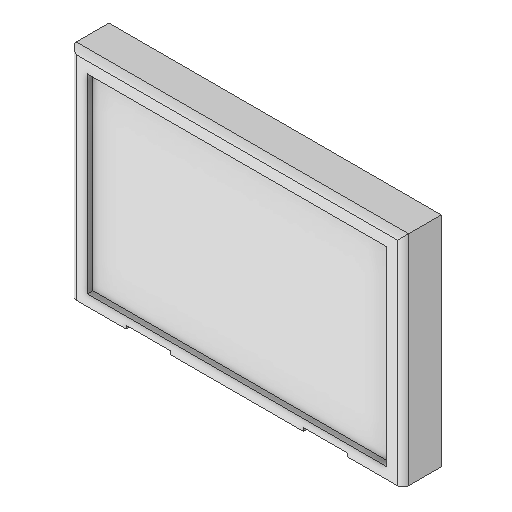
# Autodesk Inventor part: PLATE 2
Saved by Autodesk Inventor 2025.3 (Build 293356030, 356C)
## iProperties
Created: 2025-09-26
Part Number: PLATE 2
Material: 일반
Document SubType Name: Modeling
Designer: joseph
Density: 1 g/cm^3
Appearance: 기본값
Author: joseph
Autodesk Inventor part; units mm, degrees
ref_plane "YZ Plane" through (0, 0, 0) normal (1, 0, 0) x (0, 1, 0)
ref_plane "XZ Plane" through (0, 0, 0) normal (0, 1, 0) x (-1, 0, 0)
ref_plane "XY Plane" through (0, 0, 0) normal (0, 0, 1) x (1, 0, 0)
sketch "스케치1" plane through (0, 0, 0) normal (0, 0, 1) x (1, 0, 0)
  line L0 (150, 3) -> (-150, 3)
  line L1 (-150, 3) -> (-150, 200)
  line L2 (-150, 200) -> (150, 200)
  line L3 (150, 200) -> (150, 3)
  point P0 (0, 0)
  dimension "d0" = 300
  dimension "d1" = 197
  constraints: 8 end point, 2 parallel, 1 horizontal, 1 perpendicular
  measures "d0" distance of L1.end L2.end
  measures "d1" distance of L0.end L1.end
extrude "돌출1" add sketch "스케치1" along normal blind 34.5
fillet "모깎기1" radius 5 3 edges at (150, 101.5, 34.5) (-150, 101.5, 34.5) (0, 200, 34.5)
sketch "스케치2" plane through (0, 0, 0) normal (0, 0, -1) x (-1, 0, 0)
  line L0 (-150, 200) -> (150, 200) projected
  line L1 (-150, 3) -> (-150, 200) projected
  line L2 (150, 3) -> (-150, 3) projected
  line L3 (150, 200) -> (150, 3) projected
  line L4 (-147, 6) -> (-147, 197)
  line L5 (-147, 197) -> (147, 197)
  line L6 (147, 197) -> (147, 6)
  line L7 (147, 6) -> (-147, 6)
  point P0 (0, 0)
  dimension "d5" = 3
  constraints: 8 end point, 3 other
  measures "d5" distance between parallel lines of L2 L7
extrude "돌출2" cut sketch "스케치2" against normal blind 27 contours L4 L5 L6 L7
sketch "스케치3" plane through (-150, 3, 0) normal (-1, 0, 0) x (0, 0, 1)
  line L0 (29.5, 197) -> (29.5, 0) projected
  line L1 (0, 197) -> (29.5, 197) projected
  line L2 (0, 197) -> (0, 0) projected
  line L3 (0, 0) -> (29.5, 0) projected
  line L4 (9.75, 5) -> (19.75, 5)
  line L5 (19.75, 5) -> (19.75, 10)
  line L6 (19.75, 10) -> (9.75, 10)
  line L7 (9.75, 10) -> (9.75, 5)
  point P0 (0, -3)
  point P1 (14.75, 5)
  point P2 (14.75, 0)
  dimension "d8" = 10
  dimension "d9" = 5
  dimension "d10" = 5
  constraints: 8 end point, 2 midpoint, 2 parallel, 1 horizontal, 1 perpendicular, 1 vertical alignment
  measures "d8" distance of L6.end L5.end
  measures "d9" distance of L5.end L4.end
  measures "d10" distance between parallel lines of L3 L4
extrude "돌출3" cut sketch "스케치3" against normal blind 27 contours L7 L6 L5 L4
sketch "스케치4" plane through (0, 0, 34.5) normal (0, 0, 1) x (1, 0, 0)
  line L0 (145, 195) -> (145, 3) projected
  line L1 (-145, 195) -> (145, 195) projected
  line L2 (-145, 3) -> (-145, 195) projected
  line L3 (-145, 3) -> (145, 3) projected
  line L4 (-135, 185) -> (135, 185)
  line L5 (135, 185) -> (135, 13)
  line L6 (135, 13) -> (-135, 13)
  line L7 (-135, 13) -> (-135, 185)
  point P0 (0, 0)
  dimension "d13" = 10
  constraints: 8 end point, 3 other
  measures "d13" distance between parallel lines of L2 L7
extrude "돌출4" cut sketch "스케치4" against normal blind 5 contours L4 L5 L6 L7
sketch "스케치6" plane through (0, 0, 0) normal (0, 0, -1) x (-1, 0, 0)
  line L0 (-147, 197) -> (147, 197) projected
  line L1 (147, 197) -> (147, 6) projected
  line L2 (147, 6) -> (-147, 6) projected
  line L3 (-147, 6) -> (-147, 197) projected
  line L4 (-150, 200) -> (150, 200) projected
  line L5 (-150, 3) -> (-150, 200) projected
  line L6 (150, 3) -> (-150, 3) projected
  line L7 (150, 200) -> (150, 3) projected
  line L8 (-97, 147) -> (97, 147)
  line L9 (97, 147) -> (97, 56)
  line L10 (97, 56) -> (-97, 56)
  line L11 (-97, 56) -> (-97, 147)
  point P0 (0, 0)
  dimension "d16" = 50
  constraints: 8 end point, 3 other
  measures "d16" distance between parallel lines of L3 L11
extrude "돌출5" add sketch "스케치6" against normal blind 3 contours L0 L1 L2 L3
sketch "스케치7" plane through (-150, 3, 0) normal (0, -1, 0) x (1, 0, 0)
  arc A0 (300, 29.5) -> (295, 34.5) centre (295, 29.5) ccw projected
  line L0 (5, 34.5) -> (295, 34.5) projected
  arc A1 (5, 34.5) -> (0, 29.5) centre (5, 29.5) ccw projected
  line L1 (0, 0) -> (0, 29.5) projected
  line L2 (0, 0) -> (300, 0) projected
  line L3 (300, 0) -> (300, 29.5) projected
  line L4 (50, 34.5) -> (90, 34.5)
  line L5 (90, 34.5) -> (90, 18.5)
  line L6 (90, 18.5) -> (50, 18.5)
  line L7 (50, 18.5) -> (50, 34.5)
  line L8 (210, 34.5) -> (250, 34.5)
  line L9 (250, 34.5) -> (250, 18.5)
  line L10 (250, 18.5) -> (210, 18.5)
  line L11 (210, 18.5) -> (210, 34.5)
  point P0 (150, 0)
  dimension "d19" = 40
  dimension "d20" = 16
  dimension "d21" = 40
  dimension "d22" = 16
  dimension "d23" = 50
  dimension "d24" = 50
  constraints: 16 end point, 4 parallel, 2 horizontal, 2 perpendicular, 2 point on line
  measures "d19" distance of L5.end L6.end
  measures "d20" distance of L4.end L5.end
  measures "d21" distance of L9.end L10.end
  measures "d22" distance of L8.end L9.end
  measures "d23" distance from line of L7 L1.start
  measures "d24" distance from line of L3 L9.end
extrude "돌출6" cut sketch "스케치7" against normal blind 1 contours L9 L10 L11 L0 | L5 L6 L7 L0
fillet "모깎기2" radius 2 2 edges at (-80, 4, 34.5) (80, 4, 34.5) inverted yes
